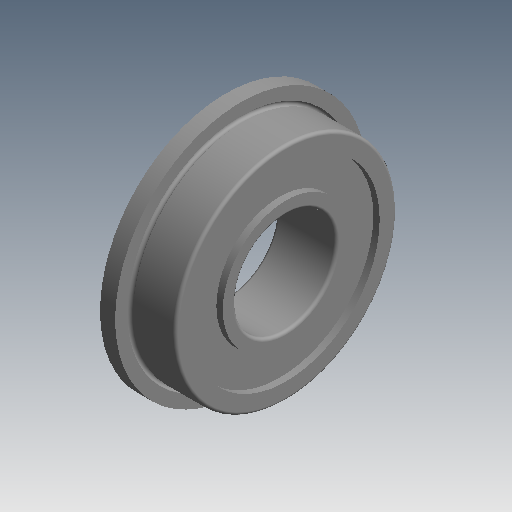
# Autodesk Inventor part: FL6900ZZ
Saved by Autodesk Inventor 2020.1 (Build 241239000, 239)
## iProperties
Part Number: FL6900ZZ
Material: 一般
Catalog Web Link: www.cadenas.de
Description: FL6 _ _ ZZ, FL6 _ _ AZZ, SFL6 _ _ ZZ, SFL6 _ _ AZZ, MFL1 _ _ ZZ, SMFL1 _ _ ZZ-Flanged Ball Bearings (Small Diameter, Deep Groove) - Double Shield Type
Vendor: MISUMI
Document SubType Name: Modeling
Designer: partserver
Manufacturer: MISUMI
Mass: 1.77032 g
Surface Area: 16.059 cm^2
Volume: 1.77032 cm^3
Density: 1 g/cm^3
Appearance: PSOLRGB-175-175-175
Category: PARTsolutions
Company: MISUMI
PSOL_IDENT_0: {$CADENAS_DATA\23d-libs\misumi\metric\12_bearing_holders\sfl608zz.prj},231 {VTYP=3D},{NB=FL6900ZZ},{
PSOL_IDENT_1: LINA=FL6900ZZ},{NN=FL6 _ _ ZZ, FL6 _ _ AZZ, SFL6 _ _ ZZ, SFL6 _ _ AZZ, MFL1 _ _ ZZ, SMFL1 _ _ ZZ},{D
PSOL_IDENT_2: ATE=09.09.2019 15:26:56},{GEOMDATE=16.08.2017 04:27:24},{VERSION=},{LINEID=170},{WBVAR=MAT},{WBNUMER
PSOL_IDENT_3: IC=}  {NB=FL6900ZZ},{LINA=FL6900ZZ},{KT=DUMMY},{PN=FL6900ZZ},{MAT=},{MAT1= '', '52100 Bearing Steel'
PSOL_IDENT_4: , 'S', '440C Stainless Steel'},{BN=6900ZZ},{DD=10.0},{AA=4.7200},{BB=1.7000},{C1=1.3000},{D=22},{B=6
PSOL_IDENT_5: .0},{D1=25.0},{C=1.5},{RR=0.30},{CR=2695},{COR=1273},{CRS=2695},{CRSS=2156},{CORS=1273},{CORSS=1018}
PSOL_IDENT_6: ,{DS=13.20},{R=0.30},{MASS=11.1},{MAT11=1},{MMMM=}
NB: FL6900ZZ
NN: FL6 _ _ ZZ, FL6 _ _ AZZ, SFL6 _ _ ZZ, SFL6 _ _ AZZ, MFL1 _ _ ZZ, SMFL1 _ _ ZZ
NT: Flanged Ball Bearings (Small Diameter, Deep Groove) - Double Shield Type
NBSYN: $PN.
LINA: FL6900ZZ
CATALOG: Misumi
PN: FL6900ZZ
MAT: 52100 Bearing Steel
BN: 6900ZZ
DD: 10
D: 22
B: 6
D1: 25
C: 1.5
RR: 0.3
CR: 2695
COR: 1273
DS: 13.2
R: 0.3
MASS: 11.1
SUPPLIER: MISUMI
ARTICLENO: FL6900ZZ
BOMINFO: FL6900ZZ
CREATOR: CADENAS GmbH
Title: FL6900ZZ
Author: Cadenas PARTsolutions
Comments: Flanged Ball Bearings (Small Diameter, Deep Groove) - Double Shield Type
Autodesk Inventor part; units mm, degrees
sketch "Sketch_1" plane through (0, 0, 0) normal (0, 0, 1) x (1, 0, 0)
  line L0 (22, 0) -> (-22, 0)
  arc A0 (0, 5.3) -> (0.3, 5) centre (0.3, 5.3) ccw
  line L1 (0.3, 5) -> (5.7, 5)
  arc A1 (5.7, 5) -> (6, 5.3) centre (5.7, 5.3) ccw
  line L2 (6, 5.3) -> (6, 6.3)
  line L3 (6, 6.3) -> (5.36, 6.3)
  line L4 (5.36, 6.3) -> (5.36, 9.3)
  line L5 (5.36, 9.3) -> (6, 9.3)
  line L6 (6, 9.3) -> (6, 12.5)
  line L7 (6, 12.5) -> (4.5, 12.5)
  line L8 (4.5, 12.5) -> (4.5, 11.3)
  arc A2 (4.2, 11) -> (4.5, 11.3) centre (4.5, 11) ccw
  line L9 (4.2, 11) -> (0.3, 11)
  arc A3 (0.3, 11) -> (0, 10.7) centre (0.3, 10.7) ccw
  line L10 (0, 10.7) -> (0, 9.3)
  line L11 (0, 9.3) -> (0.64, 9.3)
  line L12 (0.64, 9.3) -> (0.64, 6.3)
  line L13 (0.64, 6.3) -> (0, 6.3)
  line L14 (0, 6.3) -> (0, 5.3)
  constraints: 30 end point, 8 point on circle, 4 centre point
revolve "Revolution1" add sketch "Sketch_1" angle 360 about axis through (22, 0, 0) along (1, 0, 0)
ref_plane "to_housing_XY" through (0, 0, 0) normal (1, 0, 0) x (0, 0, -1)
ref_plane "to_housing_YZ" through (0, 0, 0) normal (0, 0, -1) x (0, 1, 0)
ref_plane "to_housing_ZX" through (0, 0, 0) normal (0, 1, 0) x (1, 0, 0)
body "Solid1"
